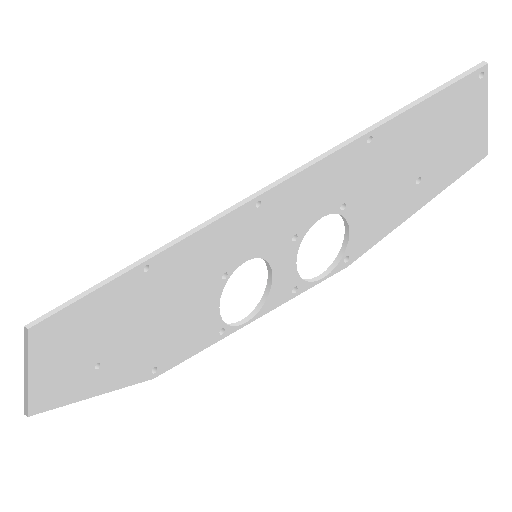
# Autodesk Inventor part: InsideChassiPlate3.0
Saved by Autodesk Inventor 2023 (Build 270158000, 158)
## iProperties
Created: 2022-09-18
Part Number: InsideChassiPlate3.0
Material: Generic
Document SubType Name: Modeling
Designer: deli
Density: 1 g/cm^3
Appearance: Default
Mass: 76.7316 g
Surface Area: 518.075 cm^2
Volume: 76.7316 cm^3
Author: deli
Autodesk Inventor part; units mm, degrees
ref_plane "YZ Plane" through (0, 0, 0) normal (1, 0, 0) x (0, 1, 0)
ref_plane "XZ Plane" through (0, 0, 0) normal (0, 1, 0) x (-1, 0, 0)
ref_plane "XY Plane" through (0, 0, 0) normal (0, 0, 1) x (1, 0, 0)
sketch "Sketch1" plane through (0, 0, 0) normal (1, 0, 0) x (0, 1, 0)
  line L0 (153.267, 5.6365) -> (153.267, -132.1707) projected
  arc A0 (153.267, -132.1707) -> (153.3544, -133.1015) centre (158.267, -132.1707) ccw projected
  line L1 (153.3544, -133.1015) -> (172.4208, -233.7253) projected
  line L2 (172.4208, -233.7253) -> (251.0603, -233.7253) projected
  line L3 (253.267, 23.7536) -> (253.267, 96.2747) projected
  line L4 (253.267, 96.2747) -> (174.6274, 96.2747) projected
  line L5 (174.6274, 96.2747) -> (153.402, 6.7905) projected
  arc A1 (153.402, 6.7905) -> (153.267, 5.6365) centre (158.267, 5.6365) ccw projected
  circle A2 centre (224.267, 11.2747) radius 2 projected
  circle A3 centre (224.267, -148.7253) radius 2 projected
  circle A4 centre (192.186, -129.5748) radius 2 projected
  circle A5 centre (158.267, -42.8128) radius 2 projected
  circle A6 centre (157.883, -94.9992) radius 2 projected
  circle A7 centre (190.1509, -94.9992) radius 2 projected
  circle A8 centre (174.017, -115.0681) radius 7 construction
  circle A9 centre (174.017, -59.9155) radius 7 construction
  circle A10 centre (181.267, -183.7253) radius 2 projected
  circle A11 centre (181.267, 46.2747) radius 2 projected
  circle A12 centre (191.6977, -44.8173) radius 2 projected
  circle A13 centre (224.267, -68.7253) radius 2 projected
  circle A14 centre (158.267, 5.6365) radius 2 projected
  circle A15 centre (158.267, -132.1707) radius 2 projected
  circle A16 centre (224.267, -228.7253) radius 2 projected
  circle A17 centre (224.267, -228.7253) radius 2 projected
  line L6 (229.267, 96.2747) -> (229.267, -233.7253)
  line L7 (525.9265, -149.4053) -> (254.1996, 22.0622) projected
  circle A18 centre (508.1, -149.9808) radius 1.5 projected
  circle A19 centre (393.9306, -77.9366) radius 1.5 projected
  circle A20 centre (279.7613, -5.8925) radius 1.5 projected
  circle A21 centre (174.017, -59.9155) radius 19
  circle A22 centre (174.017, -115.0681) radius 19
  line L8 (251.0603, -233.7253) -> (579.954, -176.0645) projected
  arc A23 (579.954, -176.0645) -> (580.5697, -168.344) centre (579.2633, -172.1246) ccw projected
  line L9 (580.5697, -168.344) -> (526.3406, -149.6042) projected
  arc A24 (525.9265, -149.4053) -> (526.3406, -149.6042) centre (526.9939, -147.7139) ccw projected
  arc A25 (253.267, 23.7536) -> (254.1996, 22.0622) centre (255.267, 23.7536) ccw projected
  circle A26 centre (579.2633, -172.1246) radius 1.6 projected
  circle A27 centre (224.267, 91.2747) radius 2 projected
  point P0 (0, 0)
  dimension "d10" = 5
  dimension "d13" = 38
  constraints: 2 centre point, 2 coincident, 2 end point, 2 point on line, 1 equal radius, 1 vertical
  measures "d10" distance from line of L6 A13.centre
  measures "d13" diameter of A21
extrude "Extrusion1" add sketch "Sketch1" along normal blind 3.175 contours A1 L5 L4 L6 L2 L1 A0 L0 | A27
body "Solid1"
